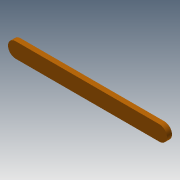
# Autodesk Inventor part: tahlo7
Saved by Autodesk Inventor 2013 (Build 170138000, 138)
## iProperties
Created: 2013-03-24
Part Number: tahlo7
Material: Generic
Document SubType Name: Modeling
Designer: idle-rug
Density: 1 g/cm^3
Author: idle-rug
Autodesk Inventor part; units mm, degrees
ref_plane "YZ Plane" through (0, 0, 0) normal (1, 0, 0) x (0, 1, 0)
ref_plane "XZ Plane" through (0, 0, 0) normal (0, 1, 0) x (-1, 0, 0)
ref_plane "XY Plane" through (0, 0, 0) normal (0, 0, 1) x (1, 0, 0)
sketch "Sketch2" plane through (0, 0, 0) normal (0, 1, 0) x (-1, 0, 0)
  line L0 (28.5, 3) -> (-28.5, 3)
  line L1 (-28.5, 3) -> (-28.5, -3)
  line L2 (-28.5, -3) -> (28.5, -3)
  line L3 (28.5, -3) -> (28.5, 3)
  line L4 (28.5, 3) -> (-28.5, -3) construction
  line L5 (-28.5, 3) -> (28.5, -3) construction
  circle A0 centre (-28.5, 0) radius 3
  circle A1 centre (28.5, 0) radius 3
  point P0 (0, 0)
  dimension "d6" = 57
  dimension "d7" = 6
  constraints: 12 end point, 4 midpoint, 2 parallel, 2 vertical alignment, 1 horizontal, 1 perpendicular, 4 other
  measures "d6" distance of L2.end L1.end
  measures "d7" distance of L1.end L0.end
extrude "Extrusion1" add sketch "Sketch2" along normal blind 2
sketch "Sketch3" plane through (0, 2, 0) normal (0, 1, 0) x (1, 0, 0)
  line L0 (-28.5, -3) -> (28.5, -3) projected
  line L1 (5, 3) -> (-5, 3)
  line L2 (-5, 3) -> (-5, -3)
  line L3 (-5, -3) -> (5, -3)
  line L4 (5, -3) -> (5, 3)
  line L5 (5, 3) -> (-5, -3) construction
  line L6 (-5, 3) -> (5, -3) construction
  point P0 (0, 0)
  dimension "d10" = 10
  constraints: 12 end point, 2 midpoint, 2 parallel, 1 horizontal, 1 perpendicular, 1 point on line
  measures "d10" distance of L3.end L2.end
extrude "Extrusion2" add sketch "Sketch3" along normal blind 7
sketch "Sketch4" plane through (0, 0, 0) normal (0, -1, 0) x (1, 0, 0)
  line L0 (-28.5, 3) -> (28.5, 3) projected
  line L1 (4, -3) -> (-4, -3)
  line L2 (-4, -3) -> (-4, 3)
  line L3 (-4, 3) -> (4, 3)
  line L4 (4, 3) -> (4, -3)
  line L5 (4, -3) -> (-4, 3) construction
  line L6 (-4, -3) -> (4, 3) construction
  point P0 (0, 0)
  dimension "d13" = 8
  constraints: 12 end point, 2 midpoint, 2 parallel, 1 horizontal, 1 perpendicular, 1 point on line
  measures "d13" distance of L2.end L3.end
extrude "Extrusion3" cut sketch "Sketch4" against normal blind 7
sketch "Sketch5" plane through (5, 2, 3) normal (1, 0, 0) x (0, 0, -1)
  line L0 (6, 0) -> (0, 0) projected
  line L1 (6, 0) -> (6, 7) projected
  line L2 (0, 7) -> (6, 7) projected
  line L3 (0, 0) -> (0, 7) projected
  point P0 (3, -2)
extrude "Extrusion4" add sketch "Sketch5" along normal blind 1
sketch "Sketch6" plane through (-5, 2, -3) normal (-1, 0, 0) x (0, 0, 1)
  line L0 (6, 0) -> (0, 0) projected
  line L1 (6, 0) -> (6, 7) projected
  line L2 (0, 7) -> (6, 7) projected
  line L3 (0, 0) -> (0, 7) projected
  point P0 (3, -2)
extrude "Extrusion5" add sketch "Sketch6" along normal blind 1
sketch "Sketch7" plane through (0, 2, 0) normal (0, 1, 0) x (1, 0, 0)
  arc A0 (28.5, -3) -> (28.5, 3) centre (28.5, 0) ccw projected
  circle A1 centre (28.5, 0) radius 1.5
  point P0 (0, 0)
  dimension "d20" = 3
  constraints: 1 centre point, 1 coincident
  measures "d20" diameter of A1
sketch "Sketch8" plane through (0, 2, 0) normal (0, 1, 0) x (1, 0, 0)
  arc A0 (-28.5, 3) -> (-28.5, -3) centre (-28.5, 0) ccw projected
  circle A1 centre (-28.5, 0) radius 1.5
  point P0 (0, 0)
  dimension "d21" = 3
  constraints: 1 centre point, 1 coincident
  measures "d21" diameter of A1
extrude "Extrusion6" cut sketch "Sketch8" against normal blind 2
extrude "Extrusion7" cut sketch "Sketch7" against normal blind 2
sketch "Sketch9" plane through (0, 9, 0) normal (0, 1, 0) x (1, 0, 0)
  line L0 (6, -3) -> (-6, -3) projected
  line L1 (6, 3) -> (6, -3) projected
  line L2 (-6, 3) -> (6, 3) projected
  line L3 (-6, -3) -> (-6, 3) projected
  point P0 (0, 0)
extrude "Extrusion8" cut sketch "Sketch9" against normal blind 7
sketch "Sketch10" plane through (-4, 0, 3) normal (1, 0, 0) x (0, 0, -1)
  line L0 (6, 2) -> (0, 2) projected
  line L1 (0, 0) -> (0, 2) projected
  line L2 (6, 0) -> (0, 0) projected
  line L3 (6, 2) -> (6, 0) projected
  point P0 (3, 0)
extrude "Extrusion9" add sketch "Sketch10" along normal blind 8
sketch "Sketch11" plane through (0, 2, 0) normal (0, 1, 0) x (1, 0, 0)
  line L0 (-28.5, 3) -> (28.5, 3) projected
  arc A0 (-28.5, 3) -> (-28.5, -3) centre (-28.5, 0) ccw projected
  line L1 (-28.5, -3) -> (28.5, -3) projected
  arc A1 (28.5, -3) -> (28.5, 3) centre (28.5, 0) ccw projected
  line L2 (4, 3) -> (-4, 3)
  line L3 (-4, 3) -> (-4, -3)
  line L4 (-4, -3) -> (4, -3)
  line L5 (4, -3) -> (4, 3)
  line L6 (4, 3) -> (-4, -3) construction
  line L7 (-4, 3) -> (4, -3) construction
  line L8 (4, 0) -> (11, 0)
  line L9 (-4, 0) -> (-11, 0)
  line L10 (-28.5, 0) -> (-11, 0)
  line L11 (28.5, 0) -> (11, 0)
  line L12 (-4, 3) -> (-11, 3)
  line L13 (-11, 3) -> (-11, -3)
  line L14 (-11, -3) -> (-4, -3)
  line L15 (-4, -3) -> (-4, 3)
  line L16 (-4, 3) -> (-11, -3) construction
  line L17 (-11, 3) -> (-4, -3) construction
  line L18 (11, 3) -> (4, 3)
  line L19 (4, 3) -> (4, -3)
  line L20 (4, -3) -> (11, -3)
  line L21 (11, -3) -> (11, 3)
  line L22 (11, 3) -> (4, -3) construction
  line L23 (4, 3) -> (11, -3) construction
  line L24 (-11, 3) -> (-28.5, 3)
  line L25 (-28.5, 3) -> (-28.5, -3)
  line L26 (-28.5, -3) -> (-11, -3)
  line L27 (-11, -3) -> (-11, 3)
  line L28 (-11, 3) -> (-28.5, -3) construction
  line L29 (-28.5, 3) -> (-11, -3) construction
  line L30 (28.5, 3) -> (11, 3)
  line L31 (11, 3) -> (11, -3)
  line L32 (11, -3) -> (28.5, -3)
  line L33 (28.5, -3) -> (28.5, 3)
  line L34 (28.5, 3) -> (11, -3) construction
  line L35 (11, 3) -> (28.5, -3) construction
  line L36 (-4, 3) -> (-4, -3)
  line L37 (-4, -3) -> (-4.01, -3)
  line L38 (-4.01, -3) -> (-4.01, 3)
  line L39 (-4.01, 3) -> (-4, 3)
  line L40 (4, 3) -> (4.01, 3)
  line L41 (4.01, 3) -> (4.01, -3)
  line L42 (4.01, -3) -> (4, -3)
  line L43 (4, -3) -> (4, 3)
  line L44 (-11, 3) -> (-11, -3)
  line L45 (-11, -3) -> (-11.01, -3)
  line L46 (-11.01, -3) -> (-11.01, 3)
  line L47 (-11.01, 3) -> (-11, 3)
  line L48 (11, 3) -> (11, -3)
  line L49 (11, -3) -> (11.01, -3)
  line L50 (11.01, -3) -> (11.01, 3)
  line L51 (11.01, 3) -> (11, 3)
  point P0 (0, 0)
  point P1 (-7.5, 0)
  point P2 (7.5, 0)
  point P3 (-19.75, 0)
  point P4 (19.75, 0)
  dimension "d32" = 8
  dimension "d33" = 7
  dimension "d34" = 7
  dimension "d35" = 17.5
  dimension "d36" = 0.01
  dimension "d37" = 6
  dimension "d38" = 0.01
  dimension "d39" = 6
  dimension "d40" = 0.01
  dimension "d41" = 6
  dimension "d42" = 0.01
  dimension "d43" = 6
  constraints: 100 end point, 16 midpoint, 13 parallel, 10 point on line, 7 perpendicular, 6 collinear, 5 horizontal
  measures "d32" distance of L4.end L3.end
  measures "d33" distance of L8.start L8.end
  measures "d34" distance of L9.start L9.end
  measures "d35" distance of L10.start L9.end
  measures "d36" distance of L14.end L37.end
  measures "d37" distance of L37.end L38.end
  measures "d38" distance of L18.end L40.end
  measures "d39" distance of L40.end L41.end
  measures "d40" distance of L26.end L45.end
  measures "d41" distance of L45.end L46.end
  measures "d42" distance of L20.end L49.end
  measures "d43" distance of L49.end L50.end
extrude "Extrusion10" cut sketch "Sketch11" against normal blind 2 contours L0 L13 L10 L46 | L10 L13 L1 L46 | L0 L3 L9 L38 | L9 L3 L1 L38 | L0 L41 L8 L5 | L8 L41 L1 L5 | L0 L50 L11 L21 | L11 L50 L1 L21
sketch "Sketch12" plane through (0, 2, 0) normal (0, 1, 0) x (1, 0, 0)
  circle A0 centre (28.5, 0) radius 1.5 projected
  arc A1 (28.5, -3) -> (28.5, 3) centre (28.5, 0) ccw projected
  circle A2 centre (28.5, 0) radius 0.005
  point P0 (0, 0)
  dimension "d46" = 0.01
  constraints: 1 centre point, 1 coincident
  measures "d46" diameter of A2
sketch "Sketch13" plane through (0, 2, 0) normal (0, 1, 0) x (1, 0, 0)
  circle A0 centre (-28.5, 0) radius 1.5 projected
  circle A1 centre (-28.5, 0) radius 0.005
  point P0 (0, 0)
  dimension "d47" = 0.01
  constraints: 1 centre point, 1 coincident
  measures "d47" diameter of A1
extrude "Extrusion11" add sketch "Sketch13" against normal blind 2
extrude "Extrusion12" add sketch "Sketch12" against normal blind 2
body "Solid1"
